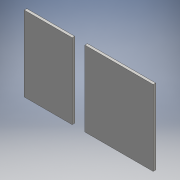
# Autodesk Inventor part: Lag1
Saved by Autodesk Inventor 2016 (Build 200138000, 138)
## iProperties
Created: 2016-12-11
Part Number: Lag1
Material: Generic
Document SubType Name: Modeling
Designer: Simon
Density: 1 g/cm^3
Appearance: Default
Author: Simon
Autodesk Inventor part; units mm, degrees
ref_plane "YZ Plane" through (0, 0, 0) normal (1, 0, 0) x (0, 1, 0)
ref_plane "XZ Plane" through (0, 0, 0) normal (0, 1, 0) x (-1, 0, 0)
ref_plane "XY Plane" through (0, 0, 0) normal (0, 0, 1) x (1, 0, 0)
sketch "Sketch2" plane through (0, 0, 0) normal (0, 1, 0) x (-1, 0, 0)
  line L0 (50.5, 29.5) -> (-50.5, 29.5)
  line L1 (-50.5, 29.5) -> (-50.5, -29.5)
  line L2 (-50.5, -29.5) -> (50.5, -29.5)
  line L3 (50.5, -29.5) -> (50.5, 29.5)
  line L4 (3, 29.5) -> (3, -29.5)
  line L5 (13, -29.5) -> (13, 29.5)
  line L6 (50.5, 0) -> (-50.5, 0)
  line L7 (3, 10.9072) -> (13, 10.9072)
  point P0 (0, 0)
  point P1 (13, 0)
  point P2 (3, 0)
  point P3 (0, 0)
  point P4 (8, 10.9072)
  dimension "d7" = 10
  dimension "d8" = 59
  dimension "d9" = 101
  dimension "d13" = 42.5
  constraints: 16 end point, 6 midpoint, 6 point on line, 4 perpendicular, 2 parallel, 1 coincident, 1 horizontal
  measures "d7" distance between parallel lines of L4 L5
  measures "d8" distance of L0.end L1.end
  measures "d9" distance of L0.start L0.end
  measures "d13" distance from line of L3 point (8, 10.907)
extrude "Extrusion2" add sketch "Sketch2" along normal blind 2 contours L3 L6 L5 L0 | L3 L2 L5 L6 | L4 L6 L1 L0 | L4 L2 L1 L6
body "Solid2"
